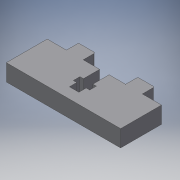
# Autodesk Inventor part: Maker_jigsaw_template
Saved by Autodesk Inventor 2019 (Build 230136000, 136)
## iProperties
Created: 2020-03-09
Part Number: Maker_jigsaw_template
Material: Generic
Document SubType Name: Modeling
Designer: Vijay
Density: 1 g/cm^3
Appearance: Default
Author: Vijay
Autodesk Inventor part; units mm, degrees
ref_plane "YZ Plane" through (0, 0, 0) normal (1, 0, 0) x (0, 1, 0)
ref_plane "XZ Plane" through (0, 0, 0) normal (0, 1, 0) x (-1, 0, 0)
ref_plane "XY Plane" through (0, 0, 0) normal (0, 0, 1) x (1, 0, 0)
sketch "Sketch1" plane through (0, 0, 0) normal (0, 1, 0) x (-1, 0, 0)
  arc A0 (32.2948, 13.759) -> (-8.6569, 13.759) centre (11.8189, 4.9346) ccw projected
  line L0 (-8.6569, 13.759) -> (-8.6569, -3.8898) projected
  line L1 (-1.7811, -3.8898) -> (-8.6569, -3.8898) projected
  line L2 (-1.7811, -3.8898) -> (-1.7811, -10.2398) projected
  line L3 (-1.7811, -10.2398) -> (4.2189, -10.2398) projected
  line L4 (4.2189, -10.2398) -> (4.2189, -3.8898) projected
  line L5 (10.3189, -3.8898) -> (4.2189, -3.8898) projected
  line L6 (10.3189, -3.8898) -> (10.3189, 2.1102) projected
  line L7 (10.3189, 2.1102) -> (9.0689, 2.1102) projected
  line L8 (9.0689, 2.1102) -> (9.0689, 4.1102) projected
  line L9 (9.0689, 4.1102) -> (10.3189, 4.1102) projected
  line L10 (10.3189, 4.1102) -> (10.3189, 6.7602) projected
  line L11 (10.3189, 6.7602) -> (13.3189, 6.7602) projected
  line L12 (13.3189, 6.7602) -> (13.3189, 4.1102) projected
  line L13 (13.3189, 4.1102) -> (14.5689, 4.1102) projected
  line L14 (14.5689, 4.1102) -> (14.5689, 2.1102) projected
  line L15 (14.5689, 2.1102) -> (13.3189, 2.1102) projected
  line L16 (13.3189, 2.1102) -> (13.3189, -3.8898) projected
  line L17 (19.4189, -3.8898) -> (13.3189, -3.8898) projected
  line L18 (19.4189, -3.8898) -> (19.4189, -10.2398) projected
  line L19 (19.4189, -10.2398) -> (25.4189, -10.2398) projected
  line L20 (25.4189, -10.2398) -> (25.4189, -3.8898) projected
  line L21 (32.2948, -3.8898) -> (25.4189, -3.8898) projected
  line L22 (32.2948, -3.8898) -> (32.2948, 13.759) projected
  circle A1 centre (11.8189, 11.3099) radius 4 projected
  line L23 (-7.9734, -40.7116) -> (-7.9734, -55.3652)
  line L24 (-1.0976, -55.3652) -> (-7.9734, -55.3652)
  line L25 (-1.0976, -55.3652) -> (-1.0976, -61.7152)
  line L26 (-1.0976, -61.7152) -> (4.9025, -61.7152)
  line L27 (4.9025, -61.7152) -> (4.9025, -55.3652)
  line L28 (11.0025, -55.3652) -> (4.9025, -55.3652)
  line L29 (11.0025, -55.3652) -> (11.0025, -49.3652)
  line L30 (11.0025, -49.3652) -> (9.7525, -49.3652)
  line L31 (9.7525, -49.3652) -> (9.7525, -47.3652)
  line L32 (9.7525, -47.3652) -> (11.0025, -47.3652)
  line L33 (11.0025, -47.3652) -> (11.0025, -44.7152)
  line L34 (11.0025, -44.7152) -> (14.0025, -44.7152)
  line L35 (14.0025, -44.7152) -> (14.0025, -47.3652)
  line L36 (14.0025, -47.3652) -> (15.2524, -47.3652)
  line L37 (15.2524, -47.3652) -> (15.2524, -49.3652)
  line L38 (15.2524, -49.3652) -> (14.0025, -49.3652)
  line L39 (14.0025, -49.3652) -> (14.0025, -55.3652)
  line L40 (20.1024, -55.3652) -> (14.0025, -55.3652)
  line L41 (20.1024, -55.3652) -> (20.1024, -61.7152)
  line L42 (20.1024, -61.7152) -> (26.1024, -61.7152)
  line L43 (26.1024, -61.7152) -> (26.1024, -55.3652)
  line L44 (32.9783, -55.3652) -> (26.1024, -55.3652)
  line L45 (32.9783, -55.3652) -> (32.9783, -40.7116)
  line L46 (32.9783, -40.7116) -> (-7.9734, -40.7116)
  point P0 (0, 0)
  point P1 (0.6835, -51.4754)
  point P2 (12.5025, -46.5408)
  constraints: 48 end point, 1 horizontal
extrude "Extrusion1" add sketch "Sketch1" along normal blind 6 contours L46 L45 L44 L43 L42 L41 L40 L39 L38 L37 L36 L35 L34 L33 L32 L31 L30 L29 L28 L27 L26 L25 L24 L23
sketch "Sketch2" plane through (0, 6, 0) normal (0, 1, 0) x (1, 0, 0)
  line L0 (-14.0025, 49.3652) -> (-14.0025, 55.3652) projected
  line L1 (-15.2524, 47.3652) -> (-15.2524, 49.3652) projected
  line L2 (-15.2524, 49.3652) -> (-14.0025, 49.3652) projected
  line L3 (-14.0025, 47.3652) -> (-15.2524, 47.3652) projected
  line L4 (-14.0025, 44.7152) -> (-14.0025, 47.3652) projected
  line L5 (-11.0025, 44.7152) -> (-14.0025, 44.7152) projected
  line L6 (-11.0025, 47.3652) -> (-11.0025, 44.7152) projected
  line L7 (-9.7525, 47.3652) -> (-11.0025, 47.3652) projected
  line L8 (-9.7525, 49.3652) -> (-9.7525, 47.3652) projected
  line L9 (-11.0025, 49.3652) -> (-9.7525, 49.3652) projected
  line L10 (-11.0025, 55.3652) -> (-11.0025, 49.3652) projected
  line L11 (-4.9025, 55.3652) -> (-11.0025, 55.3652) projected
  line L12 (-11.0025, 55.3652) -> (-14.0025, 55.3652)
  line L13 (-14.2025, 47.1652) -> (-15.4524, 47.1652)
  line L14 (-15.4524, 47.1652) -> (-15.4524, 49.5652)
  line L15 (-15.4524, 49.5652) -> (-14.2025, 49.5652)
  line L16 (-14.2025, 49.5652) -> (-14.2025, 55.5652)
  line L17 (-14.2025, 55.5652) -> (-10.8025, 55.5652)
  line L18 (-10.8025, 55.5652) -> (-10.8025, 49.5652)
  line L19 (-10.8025, 49.5652) -> (-9.5525, 49.5652)
  line L20 (-9.5525, 49.5652) -> (-9.5525, 47.1652)
  line L21 (-9.5525, 47.1652) -> (-10.8025, 47.1652)
  line L22 (-10.8025, 47.1652) -> (-10.8025, 44.5152)
  line L23 (-10.8025, 44.5152) -> (-14.2025, 44.5152)
  line L24 (-14.2025, 44.5152) -> (-14.2025, 47.1652)
  point P0 (0, 0)
  dimension "d2" = 0.2
  constraints: 26 end point, 1 collinear, 11 other
  measures "d2" distance between parallel lines of L4 L24
extrude "Extrusion2" cut sketch "Sketch2" against normal blind 25.4
sketch "Sketch3" plane through (0, 6, 0) normal (0, 1, 0) x (1, 0, 0)
  line L0 (2.9926, 65.1915) -> (-28.8734, 65.1915)
  line L1 (-28.8734, 65.1915) -> (-28.8734, 59.7152)
  line L2 (-28.8734, 59.7152) -> (2.9926, 59.7152)
  line L3 (2.9926, 59.7152) -> (2.9926, 65.1915)
  line L4 (-20.1024, 61.7152) -> (-26.1024, 61.7152) projected
  point P0 (0, 0)
  dimension "d5" = 2
  constraints: 8 end point, 2 parallel, 1 horizontal, 1 perpendicular
  measures "d5" distance between parallel lines of L2 L4
extrude "Extrusion3" cut sketch "Sketch3" against normal blind 25.4
fillet "Fillet1" radius 0.5 4 edges at (-26.1024, 3, -59.7152) (-20.1024, 3, -59.7152) (-4.9025, 3, -59.7152) (1.0976, 3, -59.7152)
body "Solid1"
